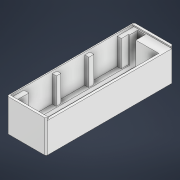
# Autodesk Inventor part: box
Saved by Autodesk Inventor 2022 (Build 260153000, 153)
## iProperties
Created: 2022-10-10
Part Number: box
Material: ABS 塑料
Document SubType Name: Modeling
Designer: 15628
Density: 1.06 g/cm^3
Appearance: 平滑 - 白色
Author: 15628
Autodesk Inventor part; units mm, degrees
ref_plane "YZ Plane" through (0, 0, 0) normal (1, 0, 0) x (0, 1, 0)
ref_plane "XZ Plane" through (0, 0, 0) normal (0, 1, 0) x (-1, 0, 0)
ref_plane "XY Plane" through (0, 0, 0) normal (0, 0, 1) x (1, 0, 0)
sketch "草图1" plane through (0, 0, 0) normal (1, 0, 0) x (0, 1, 0)
  line L0 (0, 0) -> (26, 0)
  line L1 (26, 0) -> (26, -94)
  line L2 (26, -94) -> (0, -94)
  line L3 (0, -94) -> (0, 0)
  dimension "d4" = 26
  dimension "d5" = 94
  constraints: 8 end point, 2 parallel, 1 horizontal, 1 perpendicular
  measures "d4" distance of L1.end L2.end
  measures "d5" distance of L0.end L1.end
extrude "拉伸1" add sketch "草图1" against normal blind 30
sketch "草图2" plane through (0, 26, 0) normal (0, 1, 0) x (1, 0, 0)
  line L0 (0, 0) -> (0, 94) projected
  line L1 (0, 0) -> (-1.8, 0)
  line L2 (-1.8, 0) -> (-1.8, 1.8)
  line L3 (-1.8, 1.8) -> (0, 1.8)
  line L4 (0, 1.8) -> (0, 0)
  line L5 (-30, 94) -> (-30, 0) projected
  line L6 (-30, 0) -> (-28.2, 0)
  line L7 (-28.2, 0) -> (-28.2, 1.8)
  line L8 (-28.2, 1.8) -> (-30, 1.8)
  line L9 (-30, 1.8) -> (-30, 0)
  line L10 (-30, 94) -> (-28.2, 94)
  line L11 (-28.2, 94) -> (-28.2, 92.2)
  line L12 (-28.2, 92.2) -> (-30, 92.2)
  line L13 (-30, 92.2) -> (-30, 94)
  line L14 (0, 94) -> (-1.8, 94)
  line L15 (-1.8, 94) -> (-1.8, 92.2)
  line L16 (-1.8, 92.2) -> (0, 92.2)
  line L17 (0, 92.2) -> (0, 94)
  line L18 (-28.2, 1.8) -> (-1.8, 1.8)
  line L19 (-1.8, 1.8) -> (-1.8, 92.2)
  line L20 (-1.8, 92.2) -> (-28.2, 92.2)
  line L21 (-28.2, 92.2) -> (-28.2, 1.8)
  dimension "d8" = 1.8
  dimension "d9" = 1.8
  dimension "d10" = 1.8
  dimension "d11" = 1.8
  constraints: 40 end point, 10 parallel, 5 horizontal, 5 perpendicular, 4 point on line
  measures "d8" distance of L2.end L3.end
  measures "d9" distance of L1.end L2.end
  measures "d10" distance of L8.end L7.end
  measures "d11" distance of L10.end L11.end
extrude "拉伸2" cut sketch "草图2" against normal blind 24.2 contours L18 L21 L20 L19
sketch "草图3" plane through (-28.2, 26, -1.8) normal (1, 0, 0) x (0, 0, -1)
  line L0 (0, 0) -> (0, -24.2) projected
  line L1 (92.2, 0) -> (-1.8, 0) projected
  line L2 (0, -24.2) -> (10, -24.2)
  line L3 (10, -24.2) -> (10, 0)
  line L4 (10, 0) -> (0, 0)
  line L5 (0, 0) -> (0, -24.2)
  line L6 (0, -24.2) -> (31, -24.2)
  line L7 (31, -24.2) -> (31, 0)
  line L8 (31, 0) -> (0, 0)
  line L9 (0, 0) -> (0, -24.2)
  line L10 (0, -24.2) -> (90.4, -24.2) projected
  line L11 (0, -24.2) -> (34.4, -24.2)
  line L12 (34.4, -24.2) -> (34.4, 0)
  line L13 (34.4, 0) -> (0, 0)
  line L14 (0, 0) -> (0, -24.2)
  line L15 (0, -24.2) -> (55, -24.2)
  line L16 (55, -24.2) -> (55, 0)
  line L17 (55, 0) -> (0, 0)
  line L18 (0, 0) -> (0, -24.2)
  line L19 (0, -24.2) -> (58.8, -24.2)
  line L20 (58.8, -24.2) -> (58.8, 0)
  line L21 (58.8, 0) -> (0, 0)
  line L22 (0, 0) -> (0, -24.2)
  line L23 (0, -24.2) -> (79, -24.2)
  line L24 (79, -24.2) -> (79, 0)
  line L25 (79, 0) -> (0, 0)
  line L26 (0, 0) -> (0, -24.2)
  line L27 (90.4, 0) -> (90.4, -24.2) projected
  line L28 (0, -24.2) -> (90.4, -24.2)
  line L29 (90.4, -24.2) -> (90.4, -21.2)
  line L30 (90.4, -21.2) -> (0, -21.2)
  line L31 (0, -21.2) -> (0, -24.2)
  point P0 (-1.8, -26)
  point P1 (79, -21.2)
  point P2 (58.8, -21.2)
  point P3 (55, -21.2)
  point P4 (34.4, -21.2)
  point P5 (31, -21.2)
  point P6 (10, -21.2)
  point P7 (10, -24.2)
  dimension "d14" = 10
  dimension "d15" = 31
  dimension "d16" = 34.4
  dimension "d17" = 55
  dimension "d18" = 58.8
  dimension "d19" = 79
  dimension "d20" = 3
  constraints: 56 end point, 14 parallel, 7 horizontal, 7 perpendicular, 2 point on line, 6 other
  measures "d14" distance of L4.end L3.end
  measures "d15" distance of L8.end L7.end
  measures "d16" distance of L13.end L12.end
  measures "d17" distance of L17.end L16.end
  measures "d18" distance of L21.end L20.end
  measures "d19" distance of L25.end L24.end
  measures "d20" distance of L29.end L28.end
extrude "拉伸3" add sketch "草图3" along normal blind 3 contours L1 L3 L30 L0 | L30 L3 L2 L0 | L30 L7 L6 L3 | L1 L12 L30 L7 | L30 L12 L10 L7 | L30 L16 L10 L12 | L1 L20 L30 L16 | L30 L20 L10 L16 | L30 L24 L10 L20 | L1 L27 L30 L24 | L30 L27 L10 L24
sketch "草图4" plane through (0, 1.8, 0) normal (0, 1, 0) x (1, 0, 0)
  line L0 (-1.8, 1.8) -> (-25.2, 1.8) projected
  line L1 (-25.2, 1.8) -> (-19.7, 1.8)
  line L2 (-19.7, 1.8) -> (-19.7, 53.3)
  line L3 (-20.7, 53.3) -> (-21.9, 53.3)
  line L4 (-25.2, 53.3) -> (-25.2, 1.8)
  line L5 (-19.7, 53.3) -> (-22.9, 53.3)
  line L6 (-22.9, 54.3) -> (-22.9, 62.8)
  line L7 (-21.9, 63.8) -> (-20.7, 63.8)
  line L8 (-19.7, 62.8) -> (-19.7, 54.3)
  arc A0 (-22.9, 54.3) -> (-21.9, 53.3) centre (-21.9, 54.3) ccw
  arc A1 (-21.9, 63.8) -> (-22.9, 62.8) centre (-21.9, 62.8) ccw
  arc A2 (-19.7, 62.8) -> (-20.7, 63.8) centre (-20.7, 62.8) ccw
  arc A3 (-20.7, 53.3) -> (-19.7, 54.3) centre (-20.7, 54.3) ccw
  point P0 (0, 0)
  point P1 (-22.9, 63.8)
  point P2 (-19.7, 63.8)
  dimension "d23" = 5.5
  dimension "d24" = 51.5
  dimension "d25" = 3.2
  dimension "d26" = 10.5
  dimension "d27" = 1
  constraints: 16 end point, 8 point on circle, 8 point on line, 8 tangent, 4 centre point, 4 parallel, 3 equal radius, 2 horizontal, 2 perpendicular
  measures "d23" distance of L4.start L2.end
  measures "d24" distance of L2.end L1.end
  measures "d25" distance of point (-22.9, 63.8) point (-19.7, 63.8)
  measures "d26" distance of L5.end point (-22.9, 63.8)
  measures "d27" radius of A0
extrude "拉伸4" cut sketch "草图4" against normal blind 3
sketch "草图5" plane through (0, 1.8, 0) normal (0, 1, 0) x (1, 0, 0)
  line L0 (-25.2, 92.2) -> (-25.2, 80.8) projected
  line L1 (-25.2, 92.2) -> (-23.6, 92.2)
  line L2 (-23.6, 92.2) -> (-23.6, 87.4)
  line L3 (-23.6, 87.4) -> (-25.2, 87.4)
  line L4 (-25.2, 87.4) -> (-25.2, 92.2)
  line L5 (-25.2, 92.2) -> (-1.8, 92.2) projected
  line L6 (-25.2, 92.2) -> (-22.6, 92.2)
  line L7 (-22.6, 92.2) -> (-22.6, 83.2)
  line L8 (-22.6, 83.2) -> (-25.2, 83.2)
  line L9 (-25.2, 83.2) -> (-25.2, 92.2)
  line L10 (-23.6, 87.4) -> (-22.6, 87.4)
  line L11 (-22.6, 87.4) -> (-22.6, 83.2)
  line L12 (-22.6, 83.2) -> (-23.6, 83.2)
  line L13 (-23.6, 83.2) -> (-23.6, 87.4)
  point P0 (0, 0)
  dimension "d30" = 1.6
  dimension "d31" = 4.8
  dimension "d32" = 2.6
  dimension "d33" = 9
  constraints: 24 end point, 6 parallel, 3 horizontal, 3 perpendicular
  measures "d30" distance of L2.end L3.end
  measures "d31" distance of L1.end L2.end
  measures "d32" distance of L7.end L8.end
  measures "d33" distance of L6.end L7.end
extrude "拉伸5" cut sketch "草图5" against normal blind 0.5 contours L10 L7 L8 L13
sketch "草图6" plane through (0, 1.8, 0) normal (0, 1, 0) x (1, 0, 0)
  line L0 (-25.2, 92.2) -> (-25.2, 1.8) projected
  line L1 (-25.2, 1.8) -> (-22.2, 1.8)
  line L2 (-22.2, 1.8) -> (-22.2, 46.2693)
  line L3 (-22.2, 46.2693) -> (-25.2, 46.2693)
  line L4 (-25.2, 46.2693) -> (-25.2, 1.8)
  line L5 (-22.2, 1.8) -> (-20.7, 1.8)
  line L6 (-20.7, 1.8) -> (-20.7, 12.3)
  line L7 (-20.7, 12.3) -> (-22.2, 12.3)
  line L8 (-22.2, 12.3) -> (-22.2, 1.8)
  line L9 (-22.2, 1.8) -> (-20.7, 1.8)
  line L10 (-20.7, 1.8) -> (-20.7, 15.1)
  line L11 (-20.7, 15.1) -> (-22.2, 15.1)
  line L12 (-22.2, 15.1) -> (-22.2, 1.8)
  line L13 (-22.2, 1.8) -> (-20.7, 1.8)
  line L14 (-20.7, 1.8) -> (-20.7, 21.4)
  line L15 (-20.7, 21.4) -> (-22.2, 21.4)
  line L16 (-22.2, 21.4) -> (-22.2, 1.8)
  line L17 (-22.2, 1.8) -> (-20.7, 1.8)
  line L18 (-20.7, 1.8) -> (-20.7, 24.2)
  line L19 (-20.7, 24.2) -> (-22.2, 24.2)
  line L20 (-22.2, 24.2) -> (-22.2, 1.8)
  line L21 (-22.2, 1.8) -> (-20.7, 1.8)
  line L22 (-20.7, 1.8) -> (-20.7, 30.3)
  line L23 (-20.7, 30.3) -> (-22.2, 30.3)
  line L24 (-22.2, 30.3) -> (-22.2, 1.8)
  line L25 (-22.2, 1.8) -> (-20.7, 1.8)
  line L26 (-20.7, 1.8) -> (-20.7, 33.3)
  line L27 (-20.7, 33.3) -> (-22.2, 33.3)
  line L28 (-22.2, 33.3) -> (-22.2, 1.8)
  line L29 (-22.2, 1.8) -> (-20.7, 1.8)
  line L30 (-20.7, 1.8) -> (-20.7, 39.3)
  line L31 (-20.7, 39.3) -> (-22.2, 39.3)
  line L32 (-22.2, 39.3) -> (-22.2, 1.8)
  line L33 (-22.2, 1.8) -> (-20.7, 1.8)
  line L34 (-20.7, 1.8) -> (-20.7, 42.4)
  line L35 (-20.7, 42.4) -> (-22.2, 42.4)
  line L36 (-22.2, 42.4) -> (-22.2, 1.8)
  point P0 (0, 0)
  dimension "d36" = 3
  dimension "d37" = 1.5
  dimension "d38" = 10.5
  dimension "d39" = 13.3
  dimension "d40" = 19.6
  dimension "d41" = 22.4
  dimension "d42" = 28.5
  dimension "d43" = 31.5
  dimension "d44" = 37.5
  dimension "d45" = 40.6
  constraints: 72 end point, 18 parallel, 9 horizontal, 9 perpendicular, 3 point on line
  measures "d36" distance of L3.end L2.end
  measures "d37" distance of L7.end L6.end
  measures "d38" distance of L6.end L5.end
  measures "d39" distance of L10.end L9.end
  measures "d40" distance of L14.end L13.end
  measures "d41" distance of L18.end L17.end
  measures "d42" distance of L22.end L21.end
  measures "d43" distance of L26.end L25.end
  measures "d44" distance of L30.end L29.end
  measures "d45" distance of L34.end L33.end
extrude "拉伸6" cut sketch "草图6" against normal blind 3 contours L35 L34 L31 L2 | L2 L11 L10 L7 | L27 L26 L23 L2 | L2 L19 L18 L15
sketch "草图7" plane through (-30, 0, 0) normal (-1, 0, 0) x (0, 0, 1)
  line L0 (-94, 26) -> (-94, 0) projected
  line L1 (0, 0) -> (0, 26) projected
  line L2 (-94, 26) -> (0, 26)
  line L3 (0, 26) -> (0, 0)
  line L4 (0, 0) -> (-94, 0)
  line L5 (-94, 0) -> (-94, 26)
  constraints: 8 end point, 2 parallel, 1 horizontal, 1 perpendicular
extrude "拉伸7" cut sketch "草图7" against normal blind 1
sketch "草图8" plane through (0, 0, -94) normal (0, -1, 0) x (1, 0, 0)
  line L0 (0, 0) -> (0, 94) projected
  line L1 (-29, 0) -> (-29, 94) projected
  line L2 (0, 0) -> (-29, 0)
  line L3 (-29, 0) -> (-29, 94)
  line L4 (-29, 94) -> (0, 94)
  line L5 (0, 94) -> (0, 0)
  constraints: 8 end point, 2 parallel, 1 horizontal, 1 perpendicular
extrude "拉伸8" cut sketch "草图8" against normal blind 1
sketch "草图9" plane through (-25.2, 26, -1.8) normal (1, 0, 0) x (0, 0, -1)
  line L0 (0, -24.2) -> (0, 0) projected
  line L1 (90.4, 0) -> (0, 0) projected
  line L2 (0, -24.2) -> (10, -24.2)
  line L3 (10, -24.2) -> (10, 0)
  line L4 (10, 0) -> (0, 0)
  line L5 (0, 0) -> (0, -24.2)
  line L6 (90.4, -24.2) -> (0, -24.2) projected
  line L7 (90.4, -24.2) -> (84.4, -24.2)
  line L8 (84.4, -24.2) -> (84.4, 0)
  line L9 (84.4, 0) -> (90.4, 0)
  line L10 (90.4, 0) -> (90.4, -24.2)
  point P0 (-1.8, -26)
  dimension "d52" = 10
  dimension "d53" = 6
  constraints: 16 end point, 4 parallel, 2 horizontal, 2 perpendicular, 2 point on line
  measures "d52" distance of L4.end L3.end
  measures "d53" distance of L8.end L9.end
extrude "拉伸9" add sketch "草图9" along normal blind 0.75 contours L0 L1 L3 L2 | L8 L1 L10 L6
sketch "草图10" plane through (-25.2, 26, -1.8) normal (1, 0, 0) x (0, 0, -1)
  line L0 (90.4, 0) -> (90.4, -24.2) projected
  line L1 (90.4, -24.2) -> (10, -24.2)
  line L2 (10, -24.2) -> (10, -21.2)
  line L3 (10, -21.2) -> (90.4, -21.2)
  line L4 (90.4, -21.2) -> (90.4, -24.2)
  point P0 (-1.8, -26)
  constraints: 8 end point, 2 parallel, 1 horizontal, 1 perpendicular
extrude "拉伸10" add sketch "草图10" along normal blind 0.75
sketch "草图11" plane through (-1.8, 1.8, -92.2) normal (0, 0, 1) x (1, 0, 0)
  line L0 (0, 24.2) -> (0, 0) projected
  line L1 (0, 0) -> (-9, 0)
  line L2 (-9, 0) -> (-9, 9)
  line L3 (-9, 9) -> (0, 9)
  line L4 (0, 9) -> (0, 0)
  circle A0 centre (-9, 9) radius 9
  line L5 (-22.65, 0) -> (0, 0) projected
  line L6 (0, 0) -> (-4, 0)
  line L7 (-4, 0) -> (-4, 1.5167)
  point P0 (1.8, -1.8)
  point P1 (0, 9)
  dimension "d58" = 9
  dimension "d59" = 9
  dimension "d60" = 4
  constraints: 12 end point, 2 parallel, 2 perpendicular, 2 point on circle, 1 centre point, 1 coincident, 1 horizontal, 1 point on line
  measures "d58" distance of L2.end L3.end
  measures "d59" distance of L1.end L2.end
  measures "d60" distance of L0.end L6.end
extrude "拉伸11" add sketch "草图11" along normal up to next contours L0 L1 L7 A0
sketch "草图12" plane through (-24.45, 26, -92.2) normal (0, 0, 1) x (1, 0, 0)
  line L0 (22.65, 0) -> (5.65, 0)
  line L1 (0, 0) -> (22.65, 0) projected
  line L2 (5.65, 0) -> (5.65, -24.2)
  line L3 (0, -24.2) -> (18.65, -24.2) projected
  arc A0 (18.65, -22.6833) -> (22.65, -15.2) centre (13.65, -15.2) ccw projected
  line L4 (22.65, 0) -> (22.65, -15.2) projected
  line L5 (0, 0) -> (22.65, 0) projected
  line L6 (0, 0) -> (0, -24.2) projected
  line L7 (0, -24.2) -> (18.65, -24.2) projected
  line L8 (18.65, -24.2) -> (18.65, -22.6833) projected
  point P0 (24.45, -26)
  dimension "d63" = 17
  constraints: 4 end point, 2 point on line, 1 perpendicular
  measures "d63" distance of L0.start L0.end
extrude "拉伸12" add sketch "草图12" along normal blind 7 contours L4 A0 L8 L3 L2 L0
sketch "草图13" plane through (0, 0, 0) normal (1, 0, 0) x (0, 0, -1)
  line L0 (94, 26) -> (0, 26) projected
  line L1 (94, 1) -> (94, 26) projected
  line L2 (0, 26) -> (94, 26)
  line L3 (94, 26) -> (94, 24.2)
  line L4 (94, 24.2) -> (0, 24.2)
  line L5 (0, 24.2) -> (0, 26)
  line L6 (0, 26) -> (1, 26)
  line L7 (0, 25.1) -> (0, 26)
  line L8 (94, 26) -> (93, 26)
  line L9 (94, 25.1) -> (94, 26)
  line L10 (1.8, 1.8) -> (1.8, 26) projected
  line L11 (0, 26) -> (1.8, 26)
  line L12 (1.8, 26) -> (1.8, 24.2)
  line L13 (1.8, 24.2) -> (0, 24.2)
  line L14 (0, 24.2) -> (0, 26)
  line L15 (1.8, 24.2) -> (0.9, 24.2)
  line L16 (0.9, 24.2) -> (0.9, 25.1)
  line L17 (0.9, 25.1) -> (1.8, 25.1)
  line L18 (1.8, 25.1) -> (1.8, 24.2)
  line L19 (92.2, 26) -> (92.2, 1.8) projected
  line L20 (94, 26) -> (92.2, 26)
  line L21 (92.2, 26) -> (92.2, 24.2)
  line L22 (92.2, 24.2) -> (94, 24.2)
  line L23 (94, 24.2) -> (94, 26)
  line L24 (92.2, 24.2) -> (93.1, 24.2)
  line L25 (93.1, 24.2) -> (93.1, 25.1)
  line L26 (93.1, 25.1) -> (92.2, 25.1)
  line L27 (92.2, 25.1) -> (92.2, 24.2)
  point P0 (0, 0)
  dimension "d66" = 1.8
  constraints: 48 end point, 10 parallel, 7 horizontal, 5 perpendicular, 5 point on line
  measures "d66" distance of L2.end L3.end
extrude "拉伸13" cut sketch "草图13" against normal up to surface (28.2 mm away) contours L19 L4 L10 L0 | L26 L25 L4 L19 | L10 L4 L16 L17
chamfer "倒角1" distance 1 angle 45 8 edges at (0, 13.5, 0) (0, 13.5, -94) (0, 1, -47) (-14.5, 1, 0) (-29, 13.5, 0) (-29, 13.5, -94) (-14.5, 1, -94) (-29, 1, -47)
chamfer "倒角2" distance 0.5 angle 45 24 edges at (-21.45, 1, -12.3) (-20.7, 1, -13.7) (-22.2, 1, -13.7) (-21.45, 1, -15.1) (-21.45, 1, -21.4) (-20.7, 1, -22.8) (-22.2, 1, -22.8) (-21.45, 1, -24.2) (-21.45, 1, -30.3) (-20.7, 1, -31.8) (-22.2, 1, -31.8) (-21.45, 1, -33.3) (-21.45, 1, -39.3) (-20.7, 1, -40.85) (-22.2, 1, -40.85) (-21.45, 1, -42.4) (-21.3, 1, -53.3) (-22.6071, 1, -53.5929) (-22.9, 1, -58.55) (-22.6071, 1, -63.5071) (-21.3, 1, -63.8) (-19.9929, 1, -63.5071) (-19.7, 1, -58.55) (-19.9929, 1, -53.5929)
